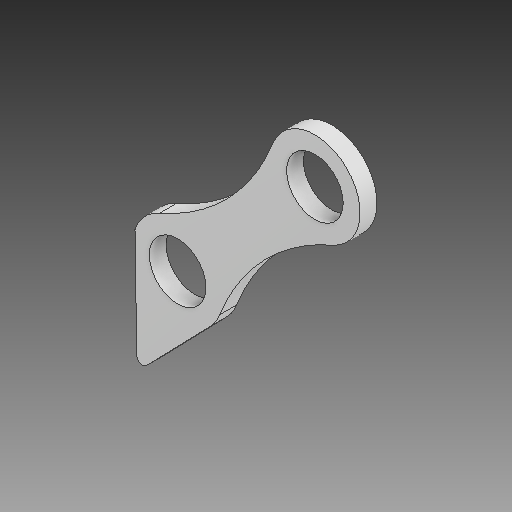
# Autodesk Inventor part: アーム揺動節2
Saved by Autodesk Inventor 2020 (Build 240168000, 168)
## iProperties
Created: 2019-09-05
Part Number: アーム揺動節2
Material: アルミニウム 2014-T4
Document SubType Name: Modeling
Designer: 雪村
Density: 2.8 g/cm^3
Appearance: サテン
Mass: 4.3893 g
Surface Area: 16.4971 cm^2
Volume: 1.56761 cm^3
Description: アルミ2000 3t
Author: 雪村
Autodesk Inventor part; units mm, degrees
ref_plane "YZ Plane" through (0, 0, 0) normal (1, 0, 0) x (0, 1, 0)
ref_plane "XZ Plane" through (0, 0, 0) normal (0, 1, 0) x (-1, 0, 0)
ref_plane "XY Plane" through (0, 0, 0) normal (0, 0, 1) x (1, 0, 0)
sketch "スケッチ2" plane through (0, 0, 0) normal (0, 0, 1) x (1, 0, 0)
  circle A0 centre (-56.644, 91.4364) radius 8.025
  circle A1 centre (-56.644, 91.4364) radius 5.025
  arc A2 (-29.1424, 109.2011) -> (-49.1672, 88.5212) centre (-14.5297, 75.0161) ccw
  arc A3 (-59.7983, 98.8155) -> (-39.7735, 119.4954) centre (-74.411, 133.0005) ccw
  circle A4 centre (-32.2967, 116.5802) radius 8.025
  circle A5 centre (-32.2967, 116.5802) radius 5.025
  line L0 (-50.8789, 85.8539) -> (-64.3562, 71.9357)
  line L1 (-64.3562, 71.9357) -> (-64.668, 91.3073)
  line L2 (-56.644, 91.4364) -> (-32.2967, 116.5802) construction
  point P0 (0, 0)
  point P1 (0, 0)
  dimension "d5" = 45
  constraints: 6 centre point, 6 end point, 6 point on circle, 2 tangent, 1 parallel, 7 other
  measures "d5" angle of L0 L1
extrude "押し出し2" add sketch "スケッチ2" along normal blind 3
fillet "フィレット2" radius 0.5 1 edges at (-64.3562, 71.9357, 1.5)
sketch "スケッチ3" plane through (0, 0, 3) normal (0, 0, 1) x (1, 0, 0)
  line L0 (-63.5165, 72.8029) -> (-50.8789, 85.8539) projected
  arc A0 (-64.3756, 73.1427) -> (-63.5165, 72.8029) centre (-63.8757, 73.1507) ccw projected
  line L1 (-64.668, 91.3073) -> (-64.3756, 73.1427) projected
  arc A1 (-59.7983, 98.8155) -> (-64.668, 91.3073) centre (-56.644, 91.4364) ccw projected
  circle A2 centre (-56.644, 91.4364) radius 5.025 projected
  arc A3 (-50.8789, 85.8539) -> (-49.1672, 88.5212) centre (-56.644, 91.4364) ccw projected
  line L2 (-64.2129, 94.1033) -> (-63.8416, 71.0319)
  point P0 (0, 0)
  point P1 (-63.8676, 72.6508)
  dimension "d9" = 0.5
  constraints: 2 end point, 1 parallel, 1 point on circle
  measures "d9" distance between parallel lines of L1 L2
extrude "押し出し3" cut sketch "スケッチ3" against normal through all
fillet "フィレット3" radius 1 1 edges at (-63.8676, 72.6508, 1.5)
